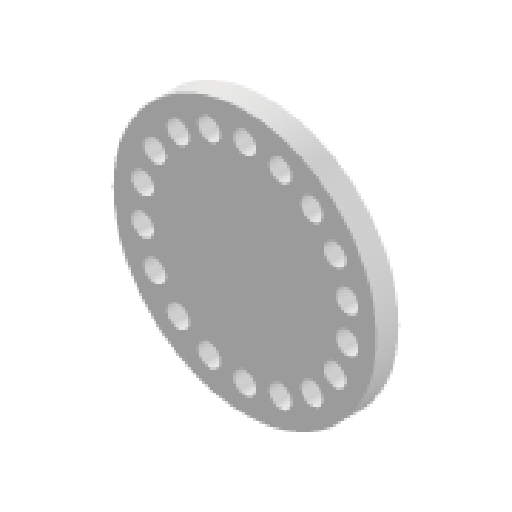
# Autodesk Inventor part: Диск
Saved by Autodesk Inventor 2026 (Build 300175000, 175)
## iProperties
Created: 2026-04-20
Part Number: Диск
Material: Типовые
Document SubType Name: Modeling
Designer: Artem Sannikov
Density: 1 g/cm^3
Appearance: По умолчанию
Author: Artem Sannikov
Autodesk Inventor part; units mm, degrees
ref_plane "YZ Plane" through (0, 0, 0) normal (1, 0, 0) x (0, 1, 0)
ref_plane "XZ Plane" through (0, 0, 0) normal (0, 1, 0) x (-1, 0, 0)
ref_plane "XY Plane" through (0, 0, 0) normal (0, 0, 1) x (1, 0, 0)
sketch "Эскиз1" plane through (0, 0, 0) normal (0, 0, 1) x (1, 0, 0)
  circle A0 centre (0, 0) radius 88.5486
  circle A1 centre (0, 0) radius 70 construction
  circle A2 centre (0, 70) radius 7.5
  circle A3 centre (0, 0) radius 70 construction
  circle A4 centre (-23.9414, 65.7785) radius 7.5
  circle A5 centre (0, 0) radius 70 construction
  circle A6 centre (-44.9951, 53.6231) radius 7.5
  circle A7 centre (0, 0) radius 70 construction
  circle A8 centre (-60.6218, 35) radius 7.5
  circle A9 centre (0, 0) radius 70 construction
  circle A10 centre (-68.9365, 12.1554) radius 7.5
  circle A11 centre (0, 0) radius 70 construction
  circle A12 centre (-68.9365, -12.1554) radius 7.5
  circle A13 centre (0, 0) radius 70 construction
  circle A14 centre (-60.6218, -35) radius 7.5
  circle A15 centre (0, 0) radius 70 construction
  circle A16 centre (-44.9951, -53.6231) radius 7.5
  circle A17 centre (0, 0) radius 70 construction
  circle A18 centre (-23.9414, -65.7785) radius 7.5
  circle A19 centre (0, 0) radius 70 construction
  circle A20 centre (0, -70) radius 7.5
  circle A21 centre (0, 0) radius 70 construction
  circle A22 centre (23.9414, -65.7785) radius 7.5
  circle A23 centre (0, 0) radius 70 construction
  circle A24 centre (44.9951, -53.6231) radius 7.5
  circle A25 centre (0, 0) radius 70 construction
  circle A26 centre (60.6218, -35) radius 7.5
  circle A27 centre (0, 0) radius 70 construction
  circle A28 centre (68.9365, -12.1554) radius 7.5
  circle A29 centre (0, 0) radius 70 construction
  circle A30 centre (68.9365, 12.1554) radius 7.5
  circle A31 centre (0, 0) radius 70 construction
  circle A32 centre (60.6218, 35) radius 7.5
  circle A33 centre (0, 0) radius 70 construction
  circle A34 centre (44.9951, 53.6231) radius 7.5
  circle A35 centre (0, 0) radius 70 construction
  circle A36 centre (23.9414, 65.7785) radius 7.5
  dimension "d0" = 140
  dimension "d1" = 15
  dimension "d4" = 360
  constraints: 19 centre point, 2 coincident, 2 vertical alignment, 125 other
  measures "d1" diameter of A2
extrude "Выдавливание1" add sketch "Эскиз1" against normal blind 15
chamfer "Фаска1" distance 2 angle 45 18 edges at (-31.4414, -65.7785, 0) (-7.5, -70, 0) (16.4414, -65.7785, 0) (37.4951, -53.6231, 0) (53.1218, -35, 0) (61.4365, -12.1554, 0) (61.4365, 12.1554, 0) (53.1218, 35, 0) (37.4951, 53.6231, 0) (16.4414, 65.7785, 0) (-7.5, 70, 0) (-31.4414, 65.7785, 0) (-52.4951, 53.6231, 0) (-68.1218, 35, 0) (-76.4365, 12.1554, 0) (-76.4365, -12.1554, 0) (-68.1218, -35, 0) (-52.4951, -53.6231, 0)
